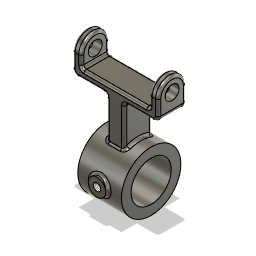
6432106821_NCV_23 (Autodesk Fusion 360 design; units mm, degrees)
Autodesk Fusion 360 part; units mm, degrees
sketch "Sketch1" plane through (0, 0, 0) normal (1, 0, 0) x (0, 0, -1)
  circle A0 centre (0, 0) radius 23
  circle A1 centre (0, 0) radius 34
  dimension "d1" = 46
  dimension "d2" = 68
  constraint coincident A0.centre A1.centre
  constraint concentric A0 A1
  measures "d1" diameter of A0
  measures "d2" diameter of A1
extrude "Extrude1" add sketch "Sketch1" along normal blind 25 and the other way blind 25
sketch "Sketch2" plane through (0, 0, 0) normal (0, 1, 0) x (1, 0, 0)
  line L0 (-10, -16, 34) -> (10, -16, 34)
  line L1 (10, -16, 34) -> (10, 16, 34)
  line L2 (10, 16, 34) -> (-10, 16, 34)
  line L3 (-10, 16, 34) -> (-10, -16, 34)
  dimension "d7" = 20
  dimension "d8" = 32
sketch "Sketch3" plane through (0, 0, 0) normal (1, 0, 0) x (0, 0, -1)
extrude "Extrude2" add sketch "Sketch2" against normal blind 5 contours L0 L1 L2 L3 in plane through (0, 34, 0) normal (0, 1, 0)
extrude "Extrude3" add 1 faces at (-3.3333, 34, -5.3333) along direction (0, 1, 0) blind 53
sketch "Sketch4" plane through (10, 0, 0) normal (1, 0, 0) x (0, 0, -1)
  arc A0 (16, 30) -> (-16, 30) centre (0, 0) ccw
  line L0 (16, 30) -> (16, 87)
  line L1 (16, 87) -> (-16, 87)
  line L2 (-16, 87) -> (-16, 30)
  line L3 (-16, 87) -> (16, 87)
  line L4 (16, 87) -> (16, 77)
  line L5 (16, 77) -> (-16, 77)
  line L6 (-16, 77) -> (-16, 87)
  dimension "d14" = 10
  constraint horizontal L3
  constraint vertical L4
  constraint horizontal L5
  constraint vertical L6
  constraint coincident L1.end L2.start
  measures "d14" distance of L1.end L5.end
sketch "Sketch5" plane through (-10, 0, 0) normal (-1, 0, 0) x (0, 0, 1)
  arc A0 (16, 30) -> (-16, 30) centre (0, 0) ccw
  line L0 (16, 30) -> (16, 87)
  line L1 (16, 87) -> (-16, 87)
  line L2 (-16, 87) -> (-16, 30)
  line L3 (-16, 87) -> (16, 87)
  line L4 (16, 87) -> (16, 77)
  line L5 (16, 77) -> (-16, 77)
  line L6 (-16, 77) -> (-16, 87)
  dimension "d15" = 10
  constraint horizontal L3
  constraint vertical L4
  constraint horizontal L5
  constraint vertical L6
  constraint coincident L1.end L2.start
  measures "d15" distance of L1.end L5.end
extrude "Extrude4" add sketch "Sketch4" along normal blind 39 contours L0 L1 L2 L3 L4 L5 L6
extrude "Extrude5" add sketch "Sketch5" along normal blind 39 contours L0 L1 L2 L3 L4 L5 L6
sketch "Sketch6" plane through (0, 87, 0) normal (0, 1, 0) x (-1, 0, 0)
  line L0 (-49, -16) -> (49, -16)
  line L1 (49, -16) -> (49, 16)
  line L2 (49, 16) -> (-49, 16)
  line L3 (-49, 16) -> (-49, -16)
  line L4 (49, -16) -> (39, -16)
  line L5 (39, -16) -> (39, 16)
  line L6 (39, 16) -> (49, 16)
  line L7 (49, 16) -> (49, -16)
  line L8 (-49, -16) -> (-39, -16)
  line L9 (-39, -16) -> (-39, 16)
  line L10 (-39, 16) -> (-49, 16)
  line L11 (-49, 16) -> (-49, -16)
  dimension "d20" = 10
  dimension "d21" = 10
  constraint horizontal L4
  constraint vertical L5
  constraint horizontal L6
  constraint vertical L7
  constraint coincident L0.end L1.start
  constraint horizontal L8
  constraint vertical L9
  constraint horizontal L10
  constraint vertical L11
  constraint coincident L0.start L3.end
  measures "d20" distance of L0.end L4.end
  measures "d21" distance of L0.start L8.end
extrude "Extrude6" add sketch "Sketch6" along normal blind 29 contours L0 L2 L3 L8 L9 L10 L11 | L0 L1 L2 L4 L5 L6 L7
sketch "Sketch7" plane through (49, 0, 0) normal (1, 0, 0) x (0, 0, -1)
  line L0 (-16, 77) -> (16, 77)
  line L1 (16, 77) -> (16, 116)
  line L2 (16, 116) -> (-16, 116)
  line L3 (-16, 116) -> (-16, 77)
  line L4 (0, 77) -> (0, 116) construction
  circle A0 centre (0, 100) radius 8
  circle A1 centre (0, 100) radius 16
  dimension "d24" = 16
  dimension "d25" = 23
  constraint midpoint L0 L4.start
  constraint midpoint L2 L4.end
  constraint coincident L4 A0.centre
  constraint concentric A0 A1
  constraint tangent L1 A1
  measures "d24" diameter of A0
  measures "d25" distance of L4.start A0.centre
extrude "Extrude7" cut sketch "Sketch7" against normal blind 293 contours L2 L3 A1 | L1 L2 A1 | A0
sketch "Sketch8" plane through (0, 0, 0) normal (0, 0, 1) x (1, 0, 0)
  circle A0 centre (0, 0) radius 10
  dimension "d28" = 20
  constraint coincident A0.centre origin
  measures "d28" diameter of A0
extrude "Extrude8" add sketch "Sketch8" along normal blind 37
delete_face "DeleteFace1" 1 faces at (9.9666, -0.8167, 7.6601)
sketch "Sketch9" plane through (0, 0, 16) normal (0, 0, 1) x (1, 0, 0)
  line L0 (49, 100) -> (39, 100)
  line L1 (39, 100) -> (39, 87)
  line L2 (39, 87) -> (-39, 87)
  line L3 (-39, 87) -> (-39, 100)
  line L4 (-39, 100) -> (-49, 100)
  line L5 (-49, 100) -> (-49, 77)
  line L6 (-49, 77) -> (-10, 77)
  line L7 (-10, 77) -> (-10, 30)
  line L8 (-10, 30) -> (10, 30)
  line L9 (10, 30) -> (10, 77)
  line L10 (10, 77) -> (49, 77)
  line L11 (49, 77) -> (49, 100)
  circle A0 centre (-43, 83) radius 6
  circle A1 centre (43, 83) radius 6
  dimension "d31" = 12
  dimension "d33" = 6
  dimension "d34" = 6
  dimension "d35" = 12
  dimension "d36" = 6
  dimension "d37" = 6
  measures "d31" diameter of A0
  measures "d33" distance of L5 A0.centre
  measures "d34" distance of L6 A0.centre
  measures "d35" diameter of A1
  measures "d36" distance of L10 A1.centre
  measures "d37" distance of L11 A1.centre
extrude "Extrude9" cut sketch "Sketch9" against normal blind 80 contours L10 L11 A1 | L5 L6 A0
fillet "Fillet1" radius 3 34 edges at (10, 53.5, 16) (10, 34, 0) (0, 30, 16) (-10, 53.5, 16) (10, 53.5, -16) (-10, 34, 0) (-10, 53.5, -16) (0, 30, -16) (-10, 77, 0) (-26.5, 77, 16) (-47.2426, 78.7574, 16) (-49, 91.5, 16) (-49, 116, 0) (-49, 91.5, -16) (-47.2426, 78.7574, -16) (-26.5, 77, -16) (0, 87, 16) (-39, 93.5, 16) (-39, 116, 0) (-39, 93.5, -16) (39, 93.5, 16) (39, 116, 0) (39, 93.5, -16) (-39, 87, 0) (39, 87, 0) (0, 87, -16) (26.5, 77, -16) (47.2426, 78.7574, -16) (49, 91.5, -16) (49, 116, 0) (49, 91.5, 16) (47.2426, 78.7574, 16) (26.5, 77, 16) (10, 77, 0)
sketch "Sketch10" plane through (0, 0, 0) normal (1, 0, 0) x (0, 0, -1)
fillet "Fillet2" radius 3 1 edges at (0, 10, 32.4962)
sketch "Sketch11" plane through (0, 0, 37) normal (0, 0, 1) x (1, 0, 0)
  arc A0 (-10, 0) -> (10, 0) centre (0, 0) ccw
  arc A1 (10, 0) -> (-10, 0) centre (0, 0) ccw
  circle A2 centre (0, 0) radius 5
  dimension "d44" = 10
  constraint concentric A0 A2
  measures "d44" diameter of A2
extrude "Extrude10" cut sketch "Sketch11" against normal blind 50 contours A2
thread "Thread1" "ISO Metric profile 10.0 M10x1.5 6H" major diameter 10.198 minor diameter 8.526 pitch 1.5 angle 60 resizes the face on face at (0.0284, 4.9999, 32.15)
